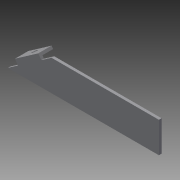
# Autodesk Inventor part: Right Forearm
Saved by Autodesk Inventor 2014 SP2 (Build 180246200, 246)
## iProperties
Created: 2015-08-01
Part Number: Right Forearm
Material: Generic
Document SubType Name: Modeling
Designer: Devon
Density: 1 g/cm^3
Appearance: Default
Author: Devon
Autodesk Inventor part; units mm, degrees
ref_plane "YZ Plane" through (0, 0, 0) normal (1, 0, 0) x (0, 1, 0)
ref_plane "XZ Plane" through (0, 0, 0) normal (0, 1, 0) x (-1, 0, 0)
ref_plane "XY Plane" through (0, 0, 0) normal (0, 0, 1) x (1, 0, 0)
sketch "Sketch1" plane through (0, 0, 0) normal (0, 0, 1) x (1, 0, 0)
  line L0 (-26.4763, -7.5222) -> (152.9112, -7.5222)
  line L1 (-26.4763, -7.5222) -> (25.5399, 28.8999)
  line L2 (-26.4763, -7.5222) -> (37.0237, -7.5222) construction
  line L3 (25.5399, 28.8999) -> (152.9112, 28.8999)
  line L4 (152.9112, 28.8999) -> (152.9112, -7.5222)
  point P0 (0, 0)
  dimension "d0" = 179.3875
  dimension "d2" = 63.5
  dimension "d3" = 35
  constraints: 10 end point, 2 horizontal, 1 equal length, 1 perpendicular
  measures "d0" distance of L0.start L0.end
  measures "d2" distance of L0.start L1.end
  measures "d3" angle of L2 L1
extrude "Extrusion1" add sketch "Sketch1" along normal blind 3.175
sketch "Sketch2" plane through (0, 0, 0) normal (0, 0, -1) x (-1, 0, 0)
  line L0 (-25.5399, 28.8999) -> (26.4763, -7.5222) projected
  line L1 (0.4682, 10.6889) -> (-13.3681, 20.3771)
  line L2 (-13.3681, 20.3771) -> (-9.7259, 25.5788)
  line L3 (-9.7259, 25.5788) -> (17.9675, 6.1876)
  line L4 (17.9675, 6.1876) -> (14.3253, 0.986)
  line L5 (14.3253, 0.986) -> (0.4682, 10.6889)
  point P0 (0, 0)
  dimension "d6" = 16.891
  dimension "d7" = 6.35
  dimension "d8" = 33.8074
  constraints: 10 end point, 2 perpendicular, 2 point on line, 1 collinear, 1 midpoint, 1 parallel
  measures "d6" distance of L1.start L1.end
  measures "d7" distance of L1.end L2.end
  measures "d8" distance of L2.end L3.end
extrude "Extrusion2" add sketch "Sketch2" against normal blind 3.175
sketch "Sketch3" plane through (0, 0, 0) normal (0, 0, -1) x (-1, 0, 0)
  line L0 (14.3253, 0.986) -> (17.9675, 6.1876) projected
  line L1 (17.9675, 6.1876) -> (-9.7259, 25.5788) projected
  line L2 (-9.7259, 25.5788) -> (-13.3681, 20.3771) projected
  line L3 (-25.5399, 28.8999) -> (-13.3681, 20.3771) projected
  line L4 (-9.7259, 25.5788) -> (17.9675, 6.1876)
  line L5 (17.9675, 6.1876) -> (16.1464, 3.5868)
  line L6 (16.1464, 3.5868) -> (-11.547, 22.9779)
  line L7 (-11.547, 22.9779) -> (-9.7259, 25.5788)
  point P0 (0, 0)
  dimension "d11" = 3.175
  constraints: 8 end point, 2 midpoint, 1 collinear, 1 parallel
  measures "d11" distance of L0.end L5.end
extrude "Extrusion3" add sketch "Sketch3" along normal blind 12.7
sketch "Sketch4" plane through (-17.9675, 6.1876, 3.175) normal (-0.5736, 0.8192, 0) x (0.8192, 0.5736, 0)
  line L0 (0, 15.875) -> (33.8074, 15.875) projected
  line L1 (16.9037, 15.875) -> (16.9037, 9.525)
  point P0 (11.1691, 3.175)
  dimension "d14" = 6.35
  constraints: 2 end point, 1 midpoint, 1 perpendicular
  measures "d14" distance of L1.start L1.end
hole "Hole1" at (-4.1208, 15.8832, -6.35) direction (0.5736, -0.8192, 0) diameter 6.35 end through all
body "Solid1"
